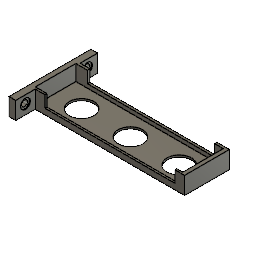
Hub v28 (Autodesk Fusion 360 design; units mm, degrees)
Autodesk Fusion 360 part; units mm, degrees
sketch "Sketch1" plane through (0, 0, 0) normal (0, 0, 1) x (1, 0, 0)
  line L0 (0, 0) -> (155, 0)
  line L1 (155, 0) -> (155, 45)
  line L2 (155, 45) -> (0, 45)
  line L3 (0, 45) -> (0, 0)
  dimension "d1" = 155
  dimension "d2" = 45
  measures "d1" distance of L0.start L0.end
  measures "d2" distance of L0.start L2.end
extrude "Extrude1" add sketch "Sketch1" along normal blind 20
sketch "Sketch2" plane through (0, 45, 0) normal (0, 1, 0) x (-1, 0, 0)
  line L0 (-155, 0) -> (0, 0)
  line L1 (0, 0) -> (0, 20)
  line L2 (0, 20) -> (-155, 20)
  line L3 (-155, 20) -> (-155, 0)
  line L4 (-155, 15) -> (-152, 15)
  line L5 (0, 10) -> (-3, 10)
  line L6 (-85.9143, 0) -> (-85.9143, 2)
  line L7 (-85.6045, 20) -> (-85.6045, 18)
  line L8 (-3, 18) -> (-151, 18)
  line L9 (-151, 18) -> (-151, 2)
  line L10 (-151, 2) -> (-3, 2)
  line L11 (-3, 2) -> (-3, 18)
  dimension "d5" = 3
  dimension "d6" = 3
  dimension "d7" = 2
  dimension "d8" = 2
  dimension "d9" = 148
  measures "d5" distance of L4.start L4.end
  measures "d6" distance of L5.start L5.end
  measures "d7" distance of L6.start L6.end
  measures "d8" distance of L7.start L7.end
  measures "d9" distance of L8.start L8.end
extrude "Extrude2" cut sketch "Sketch2" against normal blind 40 contours L8 L9 L10 L11
sketch "Sketch4" plane through (0, 0, 0) normal (0, -1, 0) x (1, 0, 0)
  line L0 (0, 0) -> (155, 0)
  line L1 (155, 0) -> (155, 20)
  line L2 (155, 20) -> (0, 20)
  line L3 (0, 20) -> (0, 0)
  line L4 (155, 10) -> (150, 10)
  line L5 (0, 10) -> (5, 10)
  line L6 (3, 2) -> (151, 2)
  line L7 (4.9248, 20) -> (4.9248, 16)
  line L8 (5.5321, 0) -> (5.5321, 4)
  line L9 (4.9248, 16) -> (149.9248, 16)
  line L10 (149.9248, 16) -> (149.9248, 4)
  line L11 (149.9248, 4) -> (4.9248, 4)
  line L12 (4.9248, 4) -> (4.9248, 16)
  dimension "d14" = 5
  dimension "d15" = 5
  dimension "d17" = 4
  dimension "d18" = 4
  dimension "d19" = 12
  dimension "d20" = 145
  measures "d14" distance of L4.start L4.end
  measures "d15" distance of L5.start L5.end
  measures "d17" distance of L7.start L7.end
  measures "d18" distance of L8.start L8.end
  measures "d19" distance of L7.end L11.end
  measures "d20" distance of L7.end L9.end
extrude "Extrude3" cut sketch "Sketch4" against normal blind 10 contours L9 L10 L11 L12
extrude "Extrude4" cut 1 faces at (3, 18.3333, 7.3333) along direction (-1, 0, 0) blind 1
extrude "Extrude5" cut 1 faces at (151, 31.6667, 12.6667) along direction (1, 0, 0) blind 1
extrude "Extrude6" cut 1 faces at (154, 45, 7.3333) along direction (0, -1, 0) blind 4
extrude "Extrude7" add 1 faces at (154, 41, 7.3333) along direction (0, 1, 0) blind 4
extrude "Extrude8" cut 1 faces at (2.9749, 5, 8) along direction (0, -1, 0) blind 2
extrude "Extrude9" cut 1 faces at (154, 45, 7.3333) along direction (0, -1, 0) blind 2
sketch "Sketch5" plane through (0, 0, 0) normal (0, 0, -1) x (-1, 0, 0)
  line L0 (0, 43) -> (-155, 43)
  line L1 (-155, 43) -> (-155, 0)
  line L2 (-155, 0) -> (0, 0)
  line L3 (0, 0) -> (0, 43)
  line L4 (0, 38.1792) -> (-5, 38.1792)
  line L5 (-5, 43) -> (-150, 43)
  line L6 (-150, 43) -> (-150, 23)
  line L7 (-150, 23) -> (-5, 23)
  line L8 (-5, 23) -> (-5, 43)
  dimension "d35" = 5
  dimension "d36" = 20
  dimension "d37" = 145
  measures "d35" distance of L4.start L4.end
  measures "d36" distance of L5.start L7.end
  measures "d37" distance of L5.start L5.end
extrude "Extrude10" cut sketch "Sketch5" against normal blind 2 contours L0 L5 L6 L7 L8
extrude "Extrude11" cut 1 faces at (101.6667, 23, 0.6667) along direction (0, -1, 0) blind 5
sketch "Sketch6" plane through (0, 0, 20) normal (0, 0, 1) x (1, 0, 0)
  line L0 (155, 43) -> (0, 43)
  line L1 (0, 43) -> (0, 0)
  line L2 (0, 0) -> (155, 0)
  line L3 (155, 0) -> (155, 43)
extrude "Extrude12" add 1 faces at (149.9248, 1, 12) along direction (-1, 0, 0) blind 5
extrude "Extrude13" add 1 faces at (4.9248, 1, 8) along direction (1, 0, 0) blind 5
extrude "Extrude14" add 1 faces at (144.9248, 1, 12) along direction (-1, 0, 0) blind 2
extrude "Extrude15" add 1 faces at (9.9248, 1, 8) along direction (1, 0, 0) blind 2
sketch "Sketch7" plane through (0, 0, 0) normal (1, 0, 0) x (0, 0, -1)
  line L0 (0, 50) -> (-20, 50)
  line L1 (-20, 50) -> (-20, -10)
  line L2 (-20, -10) -> (0, -10)
  line L3 (0, -10) -> (0, 50)
extrude "Extrude16" add sketch "Sketch7" against normal blind 15
extrude "Extrude17" add 1 faces at (-5, 50, 6.6667) along direction (0, 1, 0) blind 5
extrude "Extrude18" add 1 faces at (-5, -10, 13.3333) along direction (0, -1, 0) blind 5
extrude "Extrude19" add 1 faces at (-5, -15, 13.3333) along direction (0, -1, 0) blind 5
extrude "Extrude20" add 1 faces at (-5, 55, 6.6667) along direction (0, 1, 0) blind 8
sketch "Sketch8" plane through (0, 0, 0) normal (1, 0, 0) x (0, 0, -1)
  line L0 (-20, 43) -> (0, 43)
  line L1 (0, 43) -> (0, 63)
  line L2 (0, 63) -> (-20, 63)
  line L3 (-20, 63) -> (-20, 43)
  circle A0 centre (-10, 53) radius 1.5
  circle A1 centre (-10, 53) radius 2.5
  dimension "d60" = 3
  dimension "d61" = 5
  measures "d60" diameter of A0
  measures "d61" diameter of A1
extrude "Extrude21" cut 1 faces at (-15, 35.3333, 13.3333) along direction (1, 0, 0) blind 7
extrude "Extrude22" cut 1 faces at (-8, 35.3333, 13.3333) along direction (1, 0, 0) blind 1
extrude "Extrude23" cut sketch "Sketch8" against normal blind 1 contours A1
extrude "Extrude24" cut 1 faces at (0, 53.1166, 8.9438) along direction (-1, 0, 0) blind 7
sketch "Sketch9" plane through (0, 0, 0) normal (1, 0, 0) x (0, 0, -1)
  line L0 (0, 0) -> (-20, 0)
  line L1 (-20, 0) -> (-20, -20)
  line L2 (-20, -20) -> (0, -20)
  line L3 (0, -20) -> (0, 0)
  circle A0 centre (-10, -10) radius 1.5
  circle A1 centre (-10, -10) radius 2.5
  dimension "d70" = 3
  dimension "d71" = 5
  measures "d70" diameter of A0
  measures "d71" diameter of A1
extrude "Extrude25" cut sketch "Sketch9" against normal blind 1 contours A1
extrude "Extrude26" cut 1 faces at (0, -9.7417, 11.0902) along direction (-1, 0, 0) blind 7
extrude "Extrude27" add 1 faces at (5.3083, 3, 8) along direction (0, 1, 0) blind 40
extrude "Extrude28" cut 1 faces at (11.9248, 28.6667, 8) along direction (-1, 0, 0) blind 5
extrude "Extrude29" cut 1 faces at (142.9248, 28.6667, 12) along direction (1, 0, 0) blind 10
extrude "Extrude30" add 1 faces at (152.9248, 28.6667, 12) along direction (-1, 0, 0) blind 3
extrude "Extrude31" cut 1 faces at (6.9248, 28.6667, 8) along direction (-1, 0, 0) blind 2
extrude "Extrude32" add 1 faces at (53.3333, 26.3333, 2) along direction (0, 0, -1) blind 2
extrude "Extrude33" add 1 faces at (53.2581, 28.6667, 16) along direction (0, 0, -1) blind 12
move_body "Move1" bodies 1 to x (1, 0, 0) y (0, 0, -1) z (0, 1, 0) at (0, 44.5, 61.5)
sketch "Sketch10" plane through (0, 64.5, 0) normal (0, 1, 0) x (-1, 0, 0)
  line L0 (7, -1.5) -> (7, 81.5)
  line L1 (7, 81.5) -> (0, 81.5)
  line L2 (0, 81.5) -> (0, 61.5)
  line L3 (0, 61.5) -> (-155, 61.5)
  line L4 (-155, 61.5) -> (-155, 18.5)
  line L5 (-155, 18.5) -> (0, 18.5)
  line L6 (0, 18.5) -> (0, -1.5)
  line L7 (0, -1.5) -> (7, -1.5)
  line L8 (-148.0977, 18.5) -> (-148.0977, 20.5)
  line L9 (-148.0977, 20.5) -> (1.9023, 20.5)
  line L10 (1.9023, 20.5) -> (1.9023, 60.5)
  line L11 (1.9023, 60.5) -> (-148.0977, 60.5)
  line L12 (-148.0977, 60.5) -> (-148.0977, 20.5)
  dimension "d90" = 2
  dimension "d91" = 40
  dimension "d92" = 150
  measures "d90" distance of L8.start L8.end
  measures "d91" distance of L8.end L11.end
  measures "d92" distance of L8.end L9.end
extrude "Extrude34" add 1 faces at (51.6667, 51.1667, 61.5) along direction (0, 0, 1) blind 1
extrude "Extrude35" cut sketch "Sketch10" against normal blind 9 contours L9 L10 L11 L12
extrude "Extrude36" cut 1 faces at (98.0977, 55.5, 47.1667) along direction (0, -1, 0) blind 7
sketch "Sketch11" plane through (0, 0, 18.5) normal (0, 0, -1) x (-1, 0, 0)
  line L0 (-155, 44.5) -> (0, 44.5)
  line L1 (0, 44.5) -> (0, 64.5)
  line L2 (0, 64.5) -> (-155, 64.5)
  line L3 (-155, 64.5) -> (-155, 44.5)
  line L4 (-140.0105, 59.5304) -> (-10.0105, 59.5304)
  line L5 (-10.0105, 59.5304) -> (-10.0105, 49.5304)
  line L6 (-10.0105, 49.5304) -> (-140.0105, 49.5304)
  line L7 (-140.0105, 49.5304) -> (-140.0105, 59.5304)
  dimension "d100" = 130
  dimension "d101" = 10
  measures "d100" distance of L4.start L4.end
  measures "d101" distance of L4.start L6.end
extrude "Extrude37" cut sketch "Sketch11" against normal blind 5 contours L4 L5 L6 L7
sketch "Sketch12" plane through (0, 0, 62.5) normal (0, 0, 1) x (1, 0, 0)
  line L0 (0, 44.5) -> (155, 44.5)
  line L1 (155, 44.5) -> (155, 64.5)
  line L2 (155, 64.5) -> (0, 64.5)
  line L3 (0, 64.5) -> (0, 44.5)
  line L4 (10.0105, 59.5304) -> (150.0105, 59.5304)
  line L5 (150.0105, 59.5304) -> (150.0105, 49.5304)
  line L6 (150.0105, 49.5304) -> (10.0105, 49.5304)
  line L7 (10.0105, 49.5304) -> (10.0105, 59.5304)
  point P0 (10.0105, 59.5304)
  dimension "d104" = 140
  dimension "d105" = 10
  measures "d104" distance of P0 L4.end
  measures "d105" distance of P0 L6.end
extrude "Extrude38" cut sketch "Sketch12" against normal blind 5 contours L4 L5 L6 L7
extrude "Extrude39" add 1 faces at (150.0105, 56.197, 60.8333) along direction (-1, 0, 0) blind 7
extrude "Extrude40" cut 1 faces at (146.4019, 56.197, 57.5) along direction (0, 0, 1) blind 3
sketch "Sketch13" plane through (0, 44.5, 0) normal (0, -1, 0) x (1, 0, 0)
  line L0 (-7, 81.5) -> (-7, -1.5)
  line L1 (-7, -1.5) -> (0, -1.5)
  line L2 (0, -1.5) -> (0, 18.5)
  line L3 (0, 18.5) -> (155, 18.5)
  line L4 (155, 18.5) -> (155, 62.5)
  line L5 (155, 62.5) -> (0, 62.5)
  line L6 (0, 62.5) -> (0, 81.5)
  line L7 (0, 81.5) -> (-7, 81.5)
  circle A0 centre (25, 40) radius 12.5
  dimension "d112" = 25
  measures "d112" diameter of A0
extrude "Extrude41" cut sketch "Sketch13" against normal blind 10 contours A0
sketch "Sketch14" plane through (0, 44.5, 0) normal (0, -1, 0) x (1, 0, 0)
  circle A0 centre (25, 40) radius 12.5
  line L0 (-7, 81.5) -> (-7, -1.5)
  line L1 (-7, -1.5) -> (0, -1.5)
  line L2 (0, -1.5) -> (0, 18.5)
  line L3 (0, 18.5) -> (155, 18.5)
  line L4 (155, 18.5) -> (155, 62.5)
  line L5 (155, 62.5) -> (0, 62.5)
  line L6 (0, 62.5) -> (0, 81.5)
  line L7 (0, 81.5) -> (-7, 81.5)
  circle A1 centre (125, 40) radius 12.5
  dimension "d115" = 25
  measures "d115" diameter of A1
extrude "Extrude42" cut sketch "Sketch14" against normal blind 10 contours A1
sketch "Sketch15" plane through (0, 0, 62.5) normal (0, 0, 1) x (1, 0, 0)
  line L0 (143.0105, 49.5304) -> (10.0105, 49.5304)
  line L1 (10.0105, 49.5304) -> (10.0105, 59.5304)
  line L2 (10.0105, 59.5304) -> (143.0105, 59.5304)
  line L3 (143.0105, 59.5304) -> (143.0105, 49.5304)
  line L4 (0, 44.5) -> (155, 44.5)
  line L5 (155, 44.5) -> (155, 64.5)
  line L6 (155, 64.5) -> (0, 64.5)
  line L7 (0, 64.5) -> (0, 44.5)
  line L8 (10.0105, 59.5304) -> (10.0105, 64.5304)
  line L9 (143.0105, 59.5304) -> (143.0105, 64.5304)
  dimension "d118" = 5
  dimension "d119" = 5
  measures "d118" distance of L1.end L8.end
  measures "d119" distance of L2.end L9.end
extrude "Extrude43" cut sketch "Sketch15" against normal blind 10 contours L2 L6 L8 L9
sketch "Sketch16" plane through (0, 0, 18.5) normal (0, 0, -1) x (-1, 0, 0)
  line L0 (-10.0105, 59.5304) -> (-10.0105, 49.5304)
  line L1 (-10.0105, 49.5304) -> (-140.0105, 49.5304)
  line L2 (-140.0105, 49.5304) -> (-140.0105, 59.5304)
  line L3 (-140.0105, 59.5304) -> (-10.0105, 59.5304)
  line L4 (-155, 44.5) -> (0, 44.5)
  line L5 (0, 44.5) -> (0, 64.5)
  line L6 (0, 64.5) -> (-155, 64.5)
  line L7 (-155, 64.5) -> (-155, 44.5)
  line L8 (-140.0105, 59.5304) -> (-140.0105, 64.5304)
  line L9 (-10.0105, 59.5304) -> (-10.0105, 64.5)
  point P0 (-10.0105, 64.5)
  dimension "d122" = 5
  measures "d122" distance of L2.end L8.end
extrude "Extrude44" cut sketch "Sketch16" against normal blind 10 contours L3 L6 L8 L9
sketch "Sketch17" plane through (0, 48.5, 0) normal (0, 1, 0) x (-1, 0, 0)
  circle A0 centre (-125, 40) radius 12.5
  circle A1 centre (-25, 40) radius 12.5
  line L0 (-148.0977, 60.5) -> (-148.0977, 20.5)
  line L1 (-148.0977, 20.5) -> (1.9023, 20.5)
  line L2 (1.9023, 20.5) -> (1.9023, 60.5)
  line L3 (1.9023, 60.5) -> (-148.0977, 60.5)
  circle A2 centre (-75, 40) radius 12.5
  dimension "d125" = 25
  measures "d125" diameter of A2
extrude "Extrude45" cut sketch "Sketch17" against normal blind 10 contours A2
sketch "Sketch18" plane through (0, 0, 0) normal (1, 0, 0) x (0, 0, -1)
  circle A0 centre (-71.5, 54.5) radius 2.5
  line L0 (-62.5, 44.5) -> (-62.5, 64.5)
  line L1 (-62.5, 64.5) -> (-81.5, 64.5)
  line L2 (-81.5, 64.5) -> (-81.5, 44.5)
  line L3 (-81.5, 44.5) -> (-62.5, 44.5)
extrude "Extrude46" cut sketch "Sketch18" against normal blind 7 contours A0
sketch "Sketch19" plane through (0, 0, 0) normal (1, 0, 0) x (0, 0, -1)
  line L0 (-62.5, 44.5) -> (-62.5, 64.5)
  line L1 (-62.5, 64.5) -> (-81.5, 64.5)
  line L2 (-81.5, 64.5) -> (-81.5, 44.5)
  line L3 (-81.5, 44.5) -> (-62.5, 44.5)
extrude "Extrude47" cut 1 faces at (-2.3333, 57.8333, 81.5) along direction (0, 0, -1) blind 13
extrude "Extrude48" add 1 faces at (-2.3333, 57.8333, 68.5) along direction (0, 0, 1) blind 13
extrude "Extrude49" cut sketch "Sketch19" against normal blind 0.5
extrude "Extrude50" add 1 faces at (-0.5, 57.8333, 75.1667) along direction (1, 0, 0) blind 0.5
extrude "Extrude51" add 1 faces at (-2.3333, 57.8333, 81.5) along direction (0, 0, 1) blind 1
extrude "Extrude52" cut 1 faces at (-2.3333, 51.1667, -1.5) along direction (0, 0, 1) blind 15
extrude "Extrude53" add 1 faces at (-2.3333, 51.1667, 13.5) along direction (0, 0, -1) blind 15
sketch "Sketch20" plane through (0, 0, 0) normal (1, 0, 0) x (0, 0, -1)
  line L0 (-82.5, 44.5) -> (-62.5, 44.5)
  line L1 (-62.5, 44.5) -> (-62.5, 64.5)
  line L2 (-62.5, 64.5) -> (-82.5, 64.5)
  line L3 (-82.5, 64.5) -> (-82.5, 44.5)
  line L4 (-72.5, 64.5) -> (-72.5, 54.5)
  circle A0 centre (-72.5, 54.5) radius 3
  circle A1 centre (-72.5, 54.5) radius 5
  dimension "d144" = 10
  dimension "d145" = 6
  dimension "d146" = 10
  measures "d144" distance of L4.start L4.end
  measures "d145" diameter of A0
  measures "d146" diameter of A1
extrude "Extrude54" cut sketch "Sketch20" against normal blind 1 contours A1
extrude "Extrude55" cut 1 faces at (0, 55.4972, 71.5747) along direction (-1, 0, 0) blind 7
sketch "Sketch21" plane through (0, 0, 0) normal (1, 0, 0) x (0, 0, -1)
  line L0 (1.5, 64.5) -> (-18.5, 64.5)
  line L1 (-18.5, 64.5) -> (-18.5, 44.5)
  line L2 (-18.5, 44.5) -> (1.5, 44.5)
  line L3 (1.5, 44.5) -> (1.5, 64.5)
  line L4 (-8.9777, 64.5) -> (-8.9777, 54.5)
  circle A0 centre (-8.9777, 54.5) radius 3
  circle A1 centre (-8.9777, 54.5) radius 5
  dimension "d151" = 10
  dimension "d152" = 6
  dimension "d153" = 10
  measures "d151" distance of L4.start L4.end
  measures "d152" diameter of A0
  measures "d153" diameter of A1
extrude "Extrude56" cut sketch "Sketch21" against normal blind 2 contours A1
extrude "Extrude57" cut 1 faces at (0, 53.4675, 9.9689) along direction (-1, 0, 0) blind 7
extrude "Extrude58" add 1 faces at (-2, 54.7484, 4.663) along direction (1, 0, 0) blind 1
extrude "Extrude59" cut 1 faces at (155, 57.8333, 47.8333) along direction (-1, 0, 0) blind 4
extrude "Extrude60" cut 1 faces at (2.8985, 48.5, 40.3333) along direction (0, -1, 0) blind 2
extrude "Extrude61" cut 1 faces at (-2.3333, 64.5, 5.1667) along direction (0, -1, 0) blind 2
extrude "Extrude62" cut 1 faces at (150.0326, 64.5, 33.8333) along direction (0, -1, 0) blind 2
extrude "Extrude63" add 1 faces at (147.3368, 52.1768, 18.5) along direction (0, 0, -1) blind 1
extrude "Extrude64" cut 1 faces at (2.0686, 52.8435, 20.5) along direction (0, 0, -1) blind 1.5
extrude "Extrude65" add 1 faces at (147.3368, 52.1768, 17.5) along direction (0, 0, -1) blind 1
extrude "Extrude66" add 1 faces at (151, 50.5, 47.1667) along direction (1, 0, 0) blind 2
extrude "Extrude67" cut 1 faces at (148.0977, 57.1667, 46.6667) along direction (1, 0, 0) blind 1
extrude "Extrude68" add 1 faces at (96.6772, 49.5304, 17.3333) along direction (0, 1, 0) blind 1
extrude "Extrude69" add 1 faces at (98.6772, 49.5304, 61.8333) along direction (0, 1, 0) blind 1
